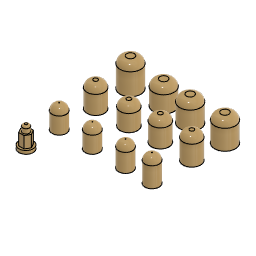
Injection mold_ (Autodesk Fusion 360 design; units mm, degrees)
Autodesk Fusion 360 part; units mm, degrees
note: some values were not read from the file. Set by a fixed rule: which sketch regions a step uses.
sketch "post body" plane through (0, 0, 0) normal (0, 0, 1) x (1, 0, 0)
  circle A0 centre (0, 0) radius 3.25
  line L0 (0, 0) -> (1.625, 2.8146)
  line L1 (0, 0) -> (-1.625, 2.8146)
  line L2 (0, 0) -> (-3.25, 0)
  line L3 (0, 0) -> (-1.625, -2.8146)
  line L4 (0, 0) -> (1.625, -2.8146)
  line L5 (1.625, -2.8146) -> (-1.625, -2.8146)
  line L6 (-1.625, -2.8146) -> (-3.25, 0)
  line L7 (-3.25, 0) -> (-1.625, 2.8146)
  line L8 (-1.625, 2.8146) -> (1.625, 2.8146)
  line L9 (0, 0) -> (3.25, 0)
  line L10 (1.625, 2.8146) -> (3.25, 0)
  line L11 (3.25, 0) -> (1.625, -2.8146)
  circle A1 centre (0, 0) radius 4.25
  dimension "d1" = 6.5
  dimension "d8" = 60
  dimension "d9" = 60
  dimension "d10" = 60
  dimension "d11" = 60
  dimension "d13" = 8.5
  constraint coincident A0.centre L0.start
  constraint coincident A0 L0.end
  constraint coincident A0 L1.end
  constraint coincident A0 L2.end
  constraint coincident A0 L3.end
  constraint coincident A0 L4.end
  constraint horizontal L9
  constraint coincident A0 L9.end
  measures "d1" diameter of A0
  measures "d8" angle of L0 L1
  measures "d9" angle of L1 L2
  measures "d10" angle of L2 L3
  measures "d11" angle of L3 L4
  measures "d13" diameter of A1
extrude "Extrude1" add sketch "post body" along normal blind 9 contours L4 L9 L11 | L0 L9 L10 | L0 L1 L8 | L3 L4 L5 | L1 L2 L7 | L2 L3 L6 makes body 1
extrude "Extrude2" add sketch "post body" along normal blind 2 contours A0 L10 | A0 L11 | A0 L8 | A0 L5 | A0 L7 | A0 L6 | A1 bodies 1
sketch "post head" plane through (0, 0, 9) normal (0, 0, 1) x (-1, 0, 0)
  line L0 (-3.25, 0) -> (-1.625, -2.8146)
  line L1 (-1.625, -2.8146) -> (1.625, -2.8146)
  line L2 (1.625, -2.8146) -> (3.25, 0)
  line L3 (3.25, 0) -> (1.625, 2.8146)
  line L4 (1.625, 2.8146) -> (-1.625, 2.8146)
  line L5 (-1.625, 2.8146) -> (-3.25, 0)
  circle A0 centre (0, 0) radius 2
  dimension "d18" = 4
  constraint coincident A0.centre origin
  measures "d18" diameter of A0
extrude "Extrude3" add sketch "post head" along normal blind 4 contours A0 bodies 1
fillet "Fillet1" radius 1.25 1 edges at (1.8647, 0.7232, 13) on bodies 1
sketch "Sketch3" plane through (0, 0, 0) normal (0, 0, 1) x (1, 0, 0)
  line L0 (0, 0) -> (-4.25, 0)
  line L1 (-4.25, 0) -> (-5.25, 0)
  line L2 (-5.25, 0) -> (-6.25, 0)
  circle A0 centre (0, 0) radius 5.25
  circle A1 centre (0, 0) radius 6.25
  dimension "d37" = 1
  dimension "d38" = 1
  constraint coincident L0.start A0.centre
  constraint horizontal L0
  constraint parallel L0 L1
  constraint parallel L1 L2
  constraint coincident L1.end A0
  constraint coincident L2.end A1
  measures "d37" distance of L0.end L1.end
  measures "d38" distance of L1.end L2.end
extrude "Extrude7" add sketch "post body" 1 faces at (1.2134, 0.1971, 0) along normal blind 14 separate body contours A0 L10 | L4 L9 L11 | L0 L9 L10 | A0 L11 | A0 L8 | L0 L1 L8 | L3 L4 L5 | A0 L5 | L1 L2 L7 | L2 L3 L6 | A0 L7 | A0 L6 | A1 on bodies 1 makes body 2
move_body "Move4" bodies 2 to x (1, 0, 0) y (0, 1, 0) z (0, 0, 1) at (0, 20, 0)
fillet "Fillet4" radius 4 1 edges at (-3.9624, 18.4631, 14) on bodies 2
extrude "Extrude8" add sketch "Sketch3" along normal blind 15 separate body contours A0 makes body 3
move_body "Move5" bodies 3 to x (1, 0, 0) y (0, 1, 0) z (0, 0, 1) at (0, 42, 0)
fillet "Fillet5" radius 4 1 edges at (-4.8947, 40.1015, 15) on bodies 3
extrude "Extrude9" add sketch "Sketch3" along normal blind 17 separate body contours A0 | A1 makes body 4
move_body "Move6" bodies 4 to x (1, 0, 0) y (0, 1, 0) z (0, 0, 1) at (0, 63, 0)
fillet "Fillet6" radius 4 1 edges at (-5.827, 60.7399, 17) on bodies 4
extrude "Extrude10" add sketch "Sketch3" along normal blind 14 separate body contours A0 makes body 5
move_body "Move7" bodies 5 to x (1, 0, 0) y (0, 1, 0) z (0, 0, 1) at (19, 43, 0)
fillet "Fillet7" radius 4 1 edges at (14.1053, 41.1015, 14) on bodies 5
extrude "Extrude11" add sketch "Sketch3" along normal blind 15 separate body contours A0 makes body 6
move_body "Move8" bodies 6 to x (1, 0, 0) y (0, 1, 0) z (0, 0, 1) at (37, 44, 0)
fillet "Fillet8" radius 4 1 edges at (32.1053, 42.1015, 15) on bodies 6
extrude "Extrude12" add sketch "Sketch3" along normal blind 16 separate body contours A0 makes body 7
move_body "Move9" bodies 7 to x (1, 0, 0) y (0, 1, 0) z (0, 0, 1) at (56, 44, 0)
fillet "Fillet9" radius 4 1 edges at (51.1053, 42.1015, 16) on bodies 7
extrude "Extrude13" add sketch "Sketch3" along normal blind 14 separate body contours A0 | A1 makes body 8
move_body "Move10" bodies 8 to x (1, 0, 0) y (0, 1, 0) z (0, 0, 1) at (19, 64, 0)
fillet "Fillet10" radius 4 1 edges at (13.173, 61.7399, 14) on bodies 8
extrude "Extrude14" add sketch "Sketch3" along normal blind 15 separate body contours A0 | A1 makes body 9
move_body "Move11" bodies 9 to x (1, 0, 0) y (0, 1, 0) z (0, 0, 1) at (36, 63, 0)
fillet "Fillet11" radius 4 1 edges at (30.173, 60.7399, 15) on bodies 9
extrude "Extrude15" add sketch "Sketch3" along normal blind 16 separate body contours A0 | A1 makes body 10
move_body "Move12" bodies 10 to x (1, 0, 0) y (0, 1, 0) z (0, 0, 1) at (57, 63, 0)
fillet "Fillet12" radius 4 1 edges at (51.173, 60.7399, 16) on bodies 10
extrude "Extrude16" add 1 faces at (1.2134, 0.1971, 0) along direction (0, 0, 1) blind 14 separate body on bodies 1 makes body 11
move_body "Move13" bodies 11 to x (1, 0, 0) y (0, 1, 0) z (0, 0, 1) at (20, 20, 0)
fillet "Fillet13" radius 4 1 edges at (16.0376, 18.4631, 14) on bodies 11
extrude "Extrude17" add 1 faces at (1.2134, 0.1971, 0) along direction (0, 0, 1) blind 15 separate body on bodies 1 makes body 12
move_body "Move14" bodies 12 to x (1, 0, 0) y (0, 1, 0) z (0, 0, 1) at (40, 20, 0)
fillet "Fillet14" radius 4 1 edges at (36.0376, 18.4631, 15) on bodies 12
extrude "Extrude18" add 1 faces at (1.2134, 0.1971, 0) along direction (0, 0, 1) blind 16 separate body on bodies 1 makes body 13
move_body "Move15" bodies 13 to x (1, 0, 0) y (0, 1, 0) z (0, 0, 1) at (56, 20, 0)
fillet "Fillet15" radius 4 1 edges at (52.0376, 18.4631, 16) on bodies 13
equation "d14 = 7 mm + 2 mm"
equation "d39 = 13.00 mm + 1 mm"
equation "d43 = 13.00 mm + 2 mm"
equation "d47 = 13.00 mm + 4 mm"
equation "d51 = 13.00 mm + 1 mm"
equation "d55 = 13.00 mm + 2 mm"
equation "d59 = 13.00 mm + 3 mm"
equation "d63 = 13.00 mm + 1 mm"
equation "d67 = 13.00 mm + 2 mm"
equation "d71 = 13.00 mm + 3 mm"
equation "d75 = -13.00 mm - 1 mm"
equation "d79 = -13.00 mm - 2 mm"
equation "d83 = -13.00 mm - 3 mm"
named bodies: "Post", "1mm body", "2mm body", "3mm body", "2mm Body +1mm", "2mm Body+2mm", "2mm Body+3mm", "3mm Body +1mm", "3mm Body +2mm", "3mm Body +3mm", "1mm Body + 1mm", "1mm Body + 2mm", "1mm Body +3mm"
